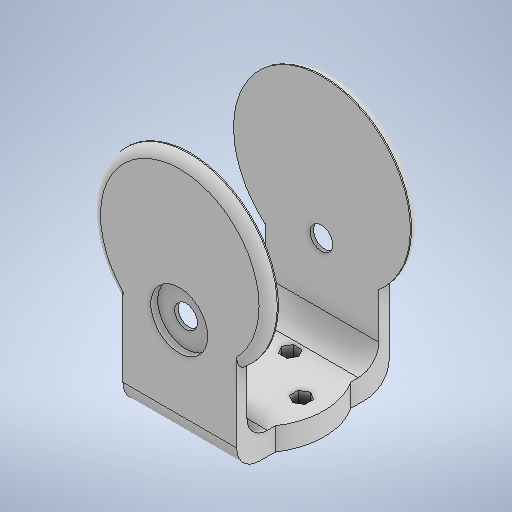
# Autodesk Inventor part: task3
Saved by Autodesk Inventor 2025.2 (Build 292293000, 293)
## iProperties
Created: 2025-07-18
Part Number: task3
Material: Generic
Document SubType Name: Modeling
Designer: PC
Density: 1 g/cm^3
Appearance: Default
Author: PC
Autodesk Inventor part; units mm, degrees
ref_plane "YZ Plane" through (0, 0, 0) normal (1, 0, 0) x (0, 1, 0)
ref_plane "XZ Plane" through (0, 0, 0) normal (0, 1, 0) x (-1, 0, 0)
sketch "Sketch1" plane through (0, 0, 0) normal (1, 0, 0) x (0, 1, 0)
  line L0 (-26.7936, -14.7843) -> (-86.7936, -14.7843)
  line L1 (-86.7936, -14.7843) -> (-86.7936, 52.2157)
  line L2 (-86.7936, 52.2157) -> (-26.8407, 52.2157)
  line L3 (-26.8407, 52.2157) -> (-26.7466, 47.7157)
  line L4 (-26.7936, -14.7843) -> (-26.7936, -10.2843)
  line L5 (-26.7936, -10.2843) -> (-76.7936, -10.2843)
  line L6 (-76.7936, -10.2843) -> (-76.7936, 47.7157)
  line L7 (-76.7936, 47.7157) -> (-26.7466, 47.7157)
  point P0 (0, 0)
  point P1 (-26.7936, -12.5343)
  point P2 (-26.7936, 49.9657)
  dimension "d0" = 4.5
  dimension "d1" = 4.5
  dimension "d4" = 60
  dimension "d5" = 50
  dimension "d9" = 58
  constraints: 16 end point, 2 horizontal, 2 midpoint, 2 perpendicular, 2 vertical, 2 vertical alignment
  measures "d0" distance of L0.start L4.end
  measures "d1" vertical distance of L2.end L3.end
  measures "d4" distance between parallel lines of L1 L4
  measures "d5" distance from line of L6 point (-26.794, -12.534)
  measures "d9" distance between parallel lines of L5 L7
extrude "Extrusion1" add sketch "Sketch1" along normal blind 50
sketch "Sketch2" plane through (0, -76.7936, 47.7157) normal (0, 1, 0) x (1, 0, 0)
  line L0 (0, 58) -> (0, 0) projected
  line L1 (0, 0) -> (50, 0) projected
  line L2 (50, 58) -> (50, 0) projected
  line L3 (0, 58) -> (50, 58) projected
  circle A0 centre (25, 29) radius 30
  point P0 (0, 47.7157)
  dimension "d12" = 60
  constraints: 1 centre point
  measures "d12" diameter of A0
fillet "Fillet1" radius 9 2 edges at (25, -76.7936, -10.2843) (25, -76.7936, 47.7157)
extrude "Extrusion2" add sketch "Sketch2" against normal blind 10 contours A0 L3 L2 L1 L0 | L0 A0 | A0 L3 | L1 A0 | A0 L2
sketch "Sketch4" plane through (0, -86.7936, -14.7843) normal (0, 0, -1) x (-1, 0, 0)
  line L0 (0, 19) -> (0, 60.047) projected
  line L1 (-50, 59.953) -> (-50, 0) projected
  line L2 (0, 29.9765) -> (-50, 29.9765)
  circle A0 centre (-25, 68.8186) radius 38.8421
  point P0 (0, 86.7936)
  point P1 (-25, 29.9765)
  constraints: 2 end point, 2 midpoint, 1 centre point, 1 perpendicular, 1 point on line, 1 tangent, 1 vertical alignment
extrude "Extrusion3" add sketch "Sketch4" against normal blind 4.5 contours A0
fillet "Fillet2" radius 4 1 edges at (25, 20.8671, -14.7843)
ref_plane "Work Plane1" through (50, -86.7936, 18.7157) normal (0, 0, -1) x (-1, 0, 0)
fillet "Fillet3" radius 10 1 edges at (25, -86.7936, -14.7843)
sketch "Sketch6" plane through (0, -86.7936, 52.2157) normal (0, 0, 1) x (1, 0, 0)
  line L0 (0, 39.0913) -> (0, 19) projected
  line L1 (50, 19) -> (0, 19) projected
  line L2 (50, 39.0913) -> (50, 19) projected
  arc A0 (50, 39.0913) -> (0, 39.0913) centre (25, 68.8186) ccw projected
  circle A1 centre (25, 68.8186) radius 38.8421
  point P0 (0, 86.7936)
  constraints: 1 centre point, 1 coincident, 1 concentric
extrude "Extrusion4" add sketch "Sketch6" against normal blind 4.5 contours A0 A1
fillet "Fillet4" radius 10 1 edges at (25, -86.7936, 52.2157)
fillet "Fillet5" radius 4 1 edges at (25, 20.8671, 52.2157)
sketch "Sketch7" plane through (25, -17.975, -14.7843) normal (0, 0, -1) x (-1, 0, 0)
  circle A0 centre (0.2258, -22.8186) radius 5
  line L0 (30, -58.8186) -> (25, -58.8186) projected
  point P0 (25, 17.975)
  dimension "d24" = 36
  dimension "d25" = 10
  constraints: 1 centre point
  measures "d24" distance from line of L0 A0.centre
  measures "d25" diameter of A0
extrude "Extrusion5" cut sketch "Sketch7" against normal through all
sketch "Sketch8" plane through (25, -17.975, -14.7843) normal (0, 0, -1) x (-1, 0, 0)
  circle A0 centre (0.2258, -22.8186) radius 5 projected
  circle A1 centre (0.2258, -22.8186) radius 12.5
  point P0 (25, 17.975)
  dimension "d28" = 25
  constraints: 1 centre point, 1 coincident
  measures "d28" diameter of A1
extrude "Extrusion6" cut sketch "Sketch8" against normal blind 3
sketch "Sketch9" plane through (0, -76.7936, 52.2157) normal (0, 0, 1) x (1, 0, 0)
  circle A0 centre (24.7742, 36) radius 5 projected
  circle A1 centre (24.7742, 36) radius 12.5 projected
  circle A2 centre (24.7742, 36) radius 12.5
  point P0 (0, 76.7936)
  constraints: 1 centre point, 1 coincident
extrude "Extrusion7" cut sketch "Sketch9" against normal blind 3
sketch "Sketch11" plane through (0, -76.7936, 38.7157) normal (0, 1, 0) x (1, 0, 0)
  line L0 (0, 3.4169) -> (0, 0) projected
  line L1 (50, 0) -> (0, 0) projected
  line L2 (50, 3.4169) -> (50, 0) projected
  arc A0 (50, 3.4169) -> (50, 36.5831) centre (25, 20) ccw projected
  line L3 (50, 40) -> (50, 36.5831) projected
  line L4 (0, 40) -> (50, 40) projected
  line L5 (0, 40) -> (0, 36.5831) projected
  arc A1 (0, 36.5831) -> (0, 3.4169) centre (25, 20) ccw projected
  line L6 (0, 40) -> (50, 40) projected
  line L7 (25, 40) -> (25, 0)
  line L8 (-5, 20) -> (55, 20)
  line L9 (26.898, 31.7126) -> (23.102, 31.7126)
  line L10 (23.102, 31.7126) -> (21.204, 35)
  line L11 (21.204, 35) -> (23.102, 38.2874)
  line L12 (23.102, 38.2874) -> (26.898, 38.2874)
  line L13 (26.898, 38.2874) -> (28.796, 35)
  line L14 (28.796, 35) -> (26.898, 31.7126)
  line L15 (48.4075, 18.0327) -> (45, 16.0654)
  line L16 (45, 16.0654) -> (41.5925, 18.0327)
  line L17 (41.5925, 18.0327) -> (41.5925, 21.9673)
  line L18 (41.5925, 21.9673) -> (45, 23.9346)
  line L19 (45, 23.9346) -> (48.4075, 21.9673)
  line L20 (48.4075, 21.9673) -> (48.4075, 18.0327)
  line L21 (26.898, 8.2874) -> (23.102, 8.2874)
  line L22 (23.102, 8.2874) -> (21.204, 5)
  line L23 (21.204, 5) -> (23.102, 1.7126)
  line L24 (23.102, 1.7126) -> (26.898, 1.7126)
  line L25 (26.898, 1.7126) -> (28.796, 5)
  line L26 (28.796, 5) -> (26.898, 8.2874)
  line L27 (1.5925, 18.0327) -> (5, 16.0654)
  line L28 (5, 16.0654) -> (8.4075, 18.0327)
  line L29 (8.4075, 18.0327) -> (8.4075, 21.9673)
  line L30 (8.4075, 21.9673) -> (5, 23.9346)
  line L31 (5, 23.9346) -> (1.5925, 21.9673)
  line L32 (1.5925, 21.9673) -> (1.5925, 18.0327)
  point P0 (0, 38.7157)
  point P1 (25, 35)
  point P2 (25, 20)
  point P3 (45, 20)
  dimension "d43" = 15
  dimension "d44" = 20
  constraints: 52 end point, 12 symmetric about line, 4 horizontal alignment, 4 midpoint, 2 point on circle, 2 point on line, 26 other
  measures "d43" distance of point (25, 20) point (25, 35)
  measures "d44" distance of point (25, 20) point (45, 20)
extrude "Extrusion9" cut sketch "Sketch11" against normal through all contours L32 L31 L30 L29 L8 | L8 L29 L28 L27 L32 | L24 L23 L22 L21 L7 | L7 L21 L26 L25 L24 | L12 L13 L14 L9 L7 | L7 L9 L10 L11 L12 | L17 L18 L19 L20 L8 | L8 L20 L15 L16 L17
body "Solid1"
